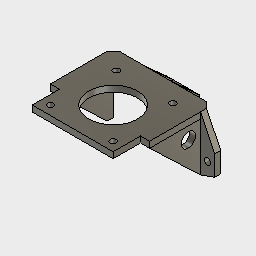
ZMotorMount (Autodesk Fusion 360 design; units mm, degrees)
Autodesk Fusion 360 part; units mm, degrees
sketch "Sketch1" plane through (0, 0, 0) normal (0, 0, 1) x (1, 0, 0)
  line L0 (0, 0) -> (-49, 0)
  line L1 (-49, 0) -> (-49, 44.5)
  line L2 (-49, 44.5) -> (0, 44.5)
  line L3 (0, 44.5) -> (0, 0)
  line L4 (0, 13.5) -> (-4.5, 13.5)
  line L5 (-4.5, 13.5) -> (-4.5, 0)
  circle A0 centre (-9, 4.5) radius 1.5
  circle A1 centre (-10.5, 35.5) radius 1.5
  circle A2 centre (-24.5, 20) radius 12
  circle A3 centre (-40, 4.5) radius 1.5
  circle A4 centre (-38.5, 35.5) radius 1.5
  line L6 (-49, 13.5) -> (-44.5, 13.5)
  line L7 (-44.5, 13.5) -> (-44.5, 0)
  line L8 (-46.112, 44.5) -> (-49, 41.62)
  line L9 (-2.8768, 44.5) -> (0, 41.62)
  dimension "d1" = 49
  dimension "d2" = 44.5
  dimension "d3" = 4.5
  dimension "d4" = 13.5
  dimension "d5" = 3
  dimension "d6" = 3
  dimension "d7" = 4.5
  dimension "d8" = 4.5
  dimension "d9" = 10.5
  dimension "d10" = 9
  dimension "d11" = 24
  dimension "d12" = 24.5
  dimension "d13" = 20
  dimension "d14" = 3
  dimension "d15" = 3
  dimension "d16" = 4.5
  dimension "d17" = 13.5
  dimension "d18" = 4.5
  dimension "d19" = 4.5
  dimension "d20" = 10.5
  dimension "d21" = 9
  dimension "d22" = 2.888
  dimension "d23" = 2.88
  dimension "d24" = 2.8768
  dimension "d25" = 2.88
  constraint horizontal L0
  constraint vertical L1
  constraint horizontal L2
  constraint vertical L3
  constraint coincident L3
  constraint coincident L0
  constraint perpendicular L0 L5
  constraint coincident L1
  constraint perpendicular L1 L6
  constraint perpendicular L6 L7
  constraint coincident L2
  measures "d4" distance of L0 L4
  measures "d5" diameter of A0
  measures "d6" diameter of A1
  measures "d7" distance of L0
  measures "d8" distance of L5
  measures "d9" distance of L3
  measures "d10" distance of L2
  measures "d11" diameter of A2
  measures "d12" distance of L1
  measures "d13" distance of L0
  measures "d14" diameter of A3
  measures "d15" diameter of A4
  measures "d18" distance of L7
  measures "d19" distance of L0
  measures "d20" distance of L1
  measures "d21" distance of L2
extrude "Extrude1" add sketch "Sketch1" along normal blind 3 contours L0 L1 L2 L3 L4 L5 L6 L7 L8 L9 makes body 1
sketch "Sketch2" plane through (0, 0, 0) normal (0, 0, -1) x (1, 0, 0)
  circle A0 centre (-9, -4.5) radius 1.5
  circle A1 centre (-24.5, -20) radius 12
  circle A2 centre (-10.5, -35.5) radius 1.5
  circle A3 centre (-40, -4.5) radius 1.5
  circle A4 centre (-38.5, -35.5) radius 1.5
  line L0 (-49, -41.62) -> (-46.112, -44.5)
  line L1 (-46.112, -44.5) -> (-2.8768, -44.5)
  line L2 (-2.8768, -44.5) -> (0, -41.62)
  line L3 (0, -41.62) -> (0, -13.5)
  line L4 (0, -13.5) -> (-4.5, -13.5)
  line L5 (-4.5, -13.5) -> (-4.5, 0)
  line L6 (-4.5, 0) -> (-44.5, 0)
  line L7 (-44.5, 0) -> (-44.5, -13.5)
  line L8 (-44.5, -13.5) -> (-49, -13.5)
  line L9 (-49, -13.5) -> (-49, -41.62)
  line L10 (-46.112, -44.5) -> (-2.8768, -44.5)
  line L11 (-49, -13.5) -> (-49, -41.62)
  line L12 (0, -41.62) -> (0, -13.5)
  line L13 (-46.112, -44.5) -> (-49, -41.62)
  line L14 (-2.8768, -44.5) -> (0, -41.62)
  line L15 (0, -41.5) -> (-49, -41.5)
  line L16 (0, -41.5) -> (49, -41.5) construction
  line L17 (-32.5, -44.5) -> (-32.5, -54.64)
  line L18 (-32.5, -44.5) -> (-21.1117, -44.5) construction
  line L19 (-32.5, -54.64) -> (-16.5, -54.64)
  line L20 (-16.5, -54.64) -> (-16.5, -44.5)
  dimension "d28" = 180
  dimension "d29" = 3
  dimension "d30" = 90
  dimension "d31" = 10.14
  dimension "d32" = 90
  dimension "d33" = 16
  dimension "d34" = 49
  dimension "d35" = 24.5
  constraint coincident L12
  constraint coincident L11
  constraint horizontal L16
  constraint coincident L10
  constraint horizontal L18
  constraint perpendicular L17 L19
  constraint coincident L18
  constraint midpoint L19
  measures "d28" angle of L15 L16
  measures "d29" distance of L1 L15
  measures "d30" angle of L17 L18
  measures "d32" angle of L18 L20
  measures "d34" distance of L3 L9
  measures "d35" distance of L9
extrude "Extrude2" add sketch "Sketch2" along normal blind 9 contours L0 L1 L2 L3 L9 L10 L11 L12 L13 L14 L15 bodies 1
sketch "Sketch3" plane through (0, 0, -9) normal (0, 0, -1) x (1, 0, 0)
  line L0 (-46.112, -44.5) -> (-2.8768, -44.5)
  line L1 (-2.8768, -44.5) -> (0, -41.62)
  line L2 (0, -41.62) -> (0, -41.5)
  line L3 (0, -41.5) -> (-49, -41.5)
  line L4 (-49, -41.5) -> (-49, -41.62)
  line L5 (-49, -41.62) -> (-46.112, -44.5)
  line L6 (-16.5, -54.64) -> (-16.5, -44.5)
  line L7 (-32.5, -54.64) -> (-16.5, -54.64)
  line L8 (-32.5, -44.5) -> (-32.5, -54.64)
  line L9 (-32.5, -44.5) -> (-21.1117, -44.5)
  line L10 (-46.112, -44.5) -> (-2.8768, -44.5)
extrude "Extrude4" add sketch "Sketch3" against normal up to surface (12 mm away) contours L0 L6 L7 L8 L9 L10 bodies 1
sketch "Sketch4" plane through (0, 54.64, 0) normal (0, 1, 0) x (-1, 0, 0)
  line L0 (32.5, 3) -> (16.5, 3)
  line L1 (16.5, 3) -> (16.5, -9)
  line L2 (16.5, -9) -> (32.5, -9)
  line L3 (32.5, -9) -> (32.5, 3)
  line L4 (32.5, -9) -> (16.5, -9)
  line L5 (16.5, -9) -> (16.5, 3)
  line L6 (32.5, -9) -> (32.5, 3)
  line L7 (32.5, 3) -> (16.5, 3)
  line L8 (16.5, -6) -> (32.5, -6)
  dimension "d41" = 3
  constraint coincident L5
  constraint coincident L6
  constraint horizontal L8
  measures "d41" distance of L2 L8
ref_plane "WorkPlane1" through (-2.8768, 44.5, 3) normal (0, 0.663814, 0.747897) x (-1, 0, 0)
sketch "Sketch5" plane through (-2.8768, 44.5, 3) normal (0, 0.663814, 0.747897) x (-1, 0, 0)
  line L0 (13, 0) -> (30.9806, 0)
  line L1 (30.9806, 0) -> (30.9806, -14.3641)
  line L2 (30.9806, -14.3641) -> (13, -14.3641)
  line L3 (13, -14.3641) -> (13, 0)
  constraint horizontal L0
  constraint vertical L1
  constraint horizontal L2
  constraint vertical L3
extrude "Extrude5" cut sketch "Sketch5" along normal blind 9 bodies 1
sketch "Sketch6" plane through (0, 0, 3) normal (0, 0, 1) x (-1, 0, 0)
  line L0 (16.5, -44.5) -> (32.5, -44.5)
  line L1 (32.5, -44.5) -> (46.112, -44.5)
  line L2 (46.112, -44.5) -> (49, -41.62)
  line L3 (49, -41.62) -> (49, -13.5)
  line L4 (49, -13.5) -> (44.5, -13.5)
  line L5 (44.5, -13.5) -> (44.5, 0)
  line L6 (44.5, 0) -> (4.5, 0)
  line L7 (4.5, 0) -> (4.5, -13.5)
  line L8 (4.5, -13.5) -> (0, -13.5)
  line L9 (0, -13.5) -> (0, -41.62)
  line L10 (0, -41.62) -> (2.8768, -44.5)
  line L11 (2.8768, -44.5) -> (16.5, -44.5)
  circle A0 centre (38.5, -35.5) radius 1.5
  circle A1 centre (40, -4.5) radius 1.5
  circle A2 centre (10.5, -35.5) radius 1.5
  circle A3 centre (24.5, -20) radius 12
  circle A4 centre (9, -4.5) radius 1.5
  line L12 (16.5, -44.5) -> (32.5, -44.5)
  line L13 (32.5, -44.5) -> (32.5, -54.64)
  line L14 (32.5, -54.64) -> (16.5, -54.64)
  line L15 (16.5, -54.64) -> (16.5, -44.5)
  line L16 (19.5, -44.5) -> (29.5, -44.5)
  line L17 (29.5, -44.5) -> (29.5, -54.64)
  line L18 (29.5, -54.64) -> (19.5, -54.64)
  line L19 (19.5, -54.64) -> (19.5, -44.5)
  dimension "d44" = 3
  dimension "d45" = 3
  constraint horizontal L16
  constraint vertical L17
  constraint horizontal L18
  constraint vertical L19
  constraint coincident L14
  constraint coincident L12
  measures "d44" distance of L13 L17
  measures "d45" distance of L15 L19
extrude "Extrude6" cut sketch "Sketch6" against normal blind 9 contours L0 L12 L14 L16 L17 L18 L19 bodies 1
sketch "Sketch7" plane through (0, 0, -9) normal (0, 0, -1) x (1, 0, 0)
  line L0 (-46.112, -44.5) -> (-32.5, -44.5)
  line L1 (-32.5, -44.5) -> (-32.5, -54.64)
  line L2 (-32.5, -54.64) -> (-16.5, -54.64)
  line L3 (-16.5, -54.64) -> (-16.5, -44.5)
  line L4 (-16.5, -44.5) -> (-2.8768, -44.5)
  line L5 (-2.8768, -44.5) -> (0, -41.62)
  line L6 (0, -41.62) -> (0, -41.5)
  line L7 (0, -41.5) -> (-49, -41.5)
  line L8 (-49, -41.5) -> (-49, -41.62)
  line L9 (-49, -41.62) -> (-46.112, -44.5)
  line L10 (0, -41.5) -> (-49, -41.5)
  line L11 (-32.5, -44.5) -> (-32.5, -54.64)
  line L12 (-16.5, -54.64) -> (-16.5, -44.5)
  circle A0 centre (-24.5, -49) radius 1.7
  dimension "d48" = 3.4
  dimension "d49" = 8
  dimension "d50" = 7.5
  measures "d48" diameter of A0
  measures "d49" distance of L1
  measures "d50" distance of L7
extrude "Extrude7" cut sketch "Sketch7" against normal up to surface (3 mm away) contours A0 bodies 1
sketch "Sketch8" plane through (0, 0, 0) normal (1, 0, 0) x (0, 1, 0)
  line L0 (41.62, -9) -> (41.62, 3)
  line L1 (41.62, 3) -> (13.5, 3)
  line L2 (13.5, 3) -> (13.5, 0)
  line L3 (13.5, 0) -> (41.5, 0)
  line L4 (41.5, 0) -> (41.5, -9)
  line L5 (41.5, -9) -> (41.62, -9)
  line L6 (13.5, 3) -> (41.62, 3)
  line L7 (13.5, 0) -> (13.5, 3)
  line L8 (41.62, 3) -> (41.62, 0)
  line L9 (41.62, 3) -> (44.62, 3) construction
  line L10 (41.62, 0) -> (41.62, -24)
  circle A0 centre (32.62, -6) radius 3.5
  line L11 (41.62, -24) -> (38.62, -24)
  line L12 (41.62, -24) -> (44.62, -24) construction
  line L13 (38.62, -24) -> (13.5, 0)
  line L14 (38.62, -24) -> (38.62, 3)
  line L15 (38.62, -24) -> (11.62, -24) construction
  dimension "d52" = 90
  dimension "d53" = 3
  dimension "d54" = 24
  dimension "d57" = 7
  dimension "d58" = 9
  dimension "d62" = 180
  dimension "d63" = 3
  dimension "d64" = 90
  dimension "d65" = 6
  constraint horizontal L9
  constraint parallel L4 L10
  constraint horizontal L12
  constraint horizontal L15
  measures "d52" angle of L8 L9
  measures "d57" diameter of A0
  measures "d58" distance of L1
  measures "d62" angle of L11 L12
  measures "d64" angle of L14 L15
  measures "d65" distance of L14
extrude "Extrude8" add sketch "Sketch8" against normal blind 2.9 contours L0 L1 L3 L4 L5 L6 L8 L10 L14 | L1 L2 L3 L6 L7 L14 bodies 1
extrude "Extrude9" cut sketch "Sketch8" against normal blind 2.9 contours A0 bodies 1
extrude "Extrude10" add sketch "Sketch8" against normal blind 2.9 separate body contours L3 L4 L5 L10 L11 L14 | L3 L13 L14 makes body 2
extrude "Extrude11" add sketch "Sketch8" along normal blind 7 separate body contours L0 L1 L3 L4 L5 L6 L8 L10 L14 | L3 L4 L5 L10 L11 L14 makes body 3
sketch "Sketch9" plane through (0, 38.62, 0) normal (0, -1, 0) x (1, 0, 0)
  line L0 (0, 3) -> (0, -24)
  line L1 (0, -24) -> (7, -24)
  line L2 (7, -24) -> (7, 3)
  line L3 (7, 3) -> (0, 3)
  line L4 (7, -11.5) -> (7, -21.5)
  line L5 (7, -11.5) -> (17, -11.5) construction
  line L6 (7, -21.5) -> (0, -24)
  line L7 (7, -11.5) -> (0, 3)
  line L8 (0, 3) -> (0, -24)
  circle A0 centre (3.5, -16.5) radius 1.6
  dimension "d70" = 90
  dimension "d71" = 10
  dimension "d72" = 14.5
  dimension "d75" = 3.2
  dimension "d76" = 3.5
  dimension "d77" = 7.5
  constraint coincident L2
  constraint horizontal L5
  measures "d70" angle of L4 L5
  measures "d72" distance of L3
  measures "d75" diameter of A0
  measures "d76" distance of L4
  measures "d77" distance of L1
extrude "Extrude12" cut sketch "Sketch9" against normal blind 3 contours L2 L3 L7 | L1 L2 L6 | A0 bodies 3
ref_plane "WorkPlane2" through (-24.5, 27.56, -3) normal (1, 0, 0) x (0, 1, 0)
mirror "Mirror1" about plane through (-24.5, 27.56, -3) normal (1, 0, 0) of bodies 2 3 makes body 4 at (-52.3052, 38.62, -7.8369) makes body 5 at (-49, 38.1633, -14.0104)
equation "d17 = d4"
equation "d18 = d8"
equation "d19 = d7"
equation "d20 = d9"
equation "d21 = d10"
equation "d25 = d23"
equation "d35 = ( 49 / 2 ) * 1 mm"
